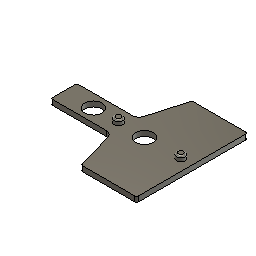
bottom_spacer (Autodesk Fusion 360 design; units mm, degrees)
Autodesk Fusion 360 part; units mm, degrees
sketch "Top" plane through (0, 0, 0) normal (0, 1, 0) x (1, 0, 0)
  line L0 (-17, 0) -> (118, 0) construction
  circle A0 centre (0, 0) radius 5
  circle A1 centre (29.5, 0) radius 5
  line L1 (-17, 7.5) -> (57, 7.5)
  line L2 (57, 7.5) -> (57, -7.5)
  line L3 (57, -7.5) -> (-17, -7.5)
  line L4 (-17, -7.5) -> (-17, 7.5)
  line L5 (57, 32) -> (25, 32)
  line L6 (25, 32) -> (25, -32)
  line L7 (25, -32) -> (57, -32)
  line L8 (57, -32) -> (57, 32)
  line L9 (25, 32) -> (18, 7.5)
  line L10 (25, -32) -> (18, -7.5)
  circle A2 centre (14.5, 0) radius 2.413
  circle A3 centre (50.5, 0) radius 2.413
  point P0 (-17, 0)
  point P1 (57, 0)
  point P2 (57, 0)
  dimension "d1" = 10
  dimension "d2" = 10
  dimension "d3" = 29.5
  dimension "d4" = 74
  dimension "d5" = 15
  dimension "d6" = 17
  dimension "d7" = 64
  dimension "d8" = 18
  dimension "d9" = 32
  dimension "d16" = 4.826
  dimension "d17" = 14.5
  dimension "d18" = 4.826
  dimension "d19" = 50.5
  constraint horizontal L0
  constraint coincident A0.centre L0
  constraint coincident A0.centre origin
  constraint coincident L0 A1.centre
  constraint horizontal L1
  constraint vertical L2
  constraint horizontal L3
  constraint vertical L4
  constraint coincident P0 L4
  constraint midpoint L4 P0
  constraint coincident L0 P0
  constraint horizontal L5
  constraint vertical L6
  constraint horizontal L7
  constraint vertical L8
  constraint midpoint L8 P2
  constraint midpoint L2 P2
  constraint coincident P2 P1
  constraint coincident L1 L9.end
  constraint symmetric L0 L5.end L6.end
  constraint symmetric L0 L9.end L10.end
  constraint coincident L0 A2.centre
  constraint midpoint L0 A3.centre
  measures "d1" diameter of A0
  measures "d2" diameter of A1
  measures "d3" distance of A0.centre A1.centre
  measures "d4" distance of L1.start L1.end
  measures "d5" distance of L1.start L3.end
  measures "d6" distance of A0.centre P0
  measures "d7" distance of L5.start L7.end
  measures "d8" horizontal distance of A0.centre L9.end
  measures "d9" distance of L5.start L5.end
  measures "d16" diameter of A2
  measures "d17" distance of A0.centre A2.centre
  measures "d18" diameter of A3
  measures "d19" distance of A0.centre A3.centre
extrude "Extrude1" add sketch "Top" along normal blind 3 contours A1 L1 L2 L3 L6 L8 | A1 L1 L3 L4 L6 | L1 L5 L6 L8 | L1 L6 L9 | L3 L6 L10 | L3 L6 L7 L8 | A2 | A3
fillet "Fillet1" radius 1 6 edges at (-17, 1.5, 7.5) (-17, 1.5, -7.5) (57, 1.5, 32) (57, 1.5, -32) (25, 1.5, -32) (25, 1.5, 32)
fillet "Fillet2" radius 4 2 edges at (18, 1.5, -7.5) (18, 1.5, 7.5)
extrude "Extrude2" add sketch "Top" along normal blind 3 from surface at 3 contours A2 | A3
fillet "Fillet3" radius 1 2 edges at (12.2503, 6, 0.8726) (48.2503, 6, 0.8726)
named bodies: "Pyxis bottom plate"
